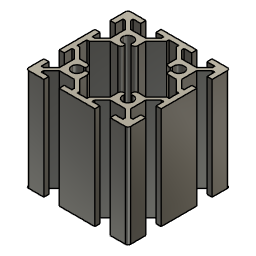
Misumi 4040 Cube (Autodesk Fusion 360 design; units mm, degrees)
Autodesk Fusion 360 part; units mm, degrees
sketch "Sketch1" plane through (0, 0, 0) normal (0, 0, 1) x (1, 0, 0)
  line L0 (-4, 2.9395) -> (-7.0605, 6)
  line L1 (-7.0605, 6) -> (-8, 6)
  line L2 (-8, 6) -> (-8, 3)
  line L3 (-8, 3) -> (-10, 3)
  line L4 (-2.9395, -4) -> (2.9395, -4)
  line L5 (-2.9395, -4) -> (-6, -7.0605)
  line L6 (-6, -7.0605) -> (-6, -8)
  line L7 (-8, -3) -> (-8, -6)
  line L8 (-8, -6) -> (-7.0608, -6)
  line L9 (-7.0608, -6) -> (-4, -2.9392)
  line L10 (-4, -2.9392) -> (-4, 2.9398)
  line L11 (-6, -8) -> (-3, -8)
  line L12 (-9, -10) -> (-3, -10)
  arc A0 (-10, -9) -> (-9, -10) centre (-9, -9) ccw
  line L13 (-10, -9) -> (-10, -3)
  line L14 (-10, -3) -> (-8, -3)
  line L15 (-3, -8) -> (-3, -10)
  line L16 (6, -7.0608) -> (2.9392, -4)
  line L17 (6, -8) -> (6, -7.0608)
  line L18 (3, -8) -> (6, -8)
  line L19 (3, -10) -> (3, -8)
  circle A1 centre (0, 0) radius 2.1
  line L20 (17.0605, -4) -> (14, -7.0605)
  line L21 (14, -7.0605) -> (14, -8)
  line L22 (17, -8) -> (17, -10)
  line L23 (14, -8) -> (17, -8)
  line L24 (24, -2.9395) -> (24, 2.9395)
  line L25 (24, -2.9395) -> (27.0605, -6)
  line L26 (27.0605, -6) -> (28, -6)
  line L27 (28, -6) -> (28, -3)
  line L28 (28, -3) -> (30, -3)
  line L29 (30, -9) -> (30, -3)
  arc A2 (29, -10) -> (30, -9) centre (29, -9) ccw
  line L30 (29, -10) -> (23, -10)
  line L31 (23, -10) -> (23, -8)
  line L32 (23, -8) -> (26, -8)
  line L33 (26, -8) -> (26, -7.0608)
  line L34 (26, -7.0608) -> (22.9392, -4)
  line L35 (22.9392, -4) -> (17.0602, -4)
  line L36 (30, 3) -> (28, 3)
  line L37 (28, 3) -> (28, 6)
  line L38 (28, 6) -> (27.0608, 6)
  line L39 (27.0608, 6) -> (24, 2.9392)
  line L40 (24, 17.0605) -> (27.0605, 14)
  line L41 (27.0605, 14) -> (28, 14)
  line L42 (28, 17) -> (30, 17)
  line L43 (28, 14) -> (28, 17)
  line L44 (22.9395, 24) -> (17.0605, 24)
  line L45 (22.9395, 24) -> (26, 27.0605)
  line L46 (26, 27.0605) -> (26, 28)
  line L47 (26, 28) -> (23, 28)
  line L48 (23, 28) -> (23, 30)
  line L49 (29, 30) -> (23, 30)
  arc A3 (30, 29) -> (29, 30) centre (29, 29) ccw
  line L50 (30, 29) -> (30, 23)
  line L51 (30, 23) -> (28, 23)
  line L52 (28, 23) -> (28, 26)
  line L53 (28, 26) -> (27.0608, 26)
  line L54 (27.0608, 26) -> (24, 22.9392)
  line L55 (24, 22.9392) -> (24, 17.0602)
  line L56 (17, 30) -> (17, 28)
  line L57 (17, 28) -> (14, 28)
  line L58 (14, 28) -> (14, 27.0608)
  line L59 (14, 27.0608) -> (17.0608, 24)
  line L60 (2.9395, 24) -> (6, 27.0605)
  line L61 (6, 27.0605) -> (6, 28)
  line L62 (3, 28) -> (3, 30)
  line L63 (6, 28) -> (3, 28)
  line L64 (-4, 22.9395) -> (-4, 17.0605)
  line L65 (-4, 22.9395) -> (-7.0605, 26)
  line L66 (-7.0605, 26) -> (-8, 26)
  line L67 (-8, 26) -> (-8, 23)
  line L68 (-8, 23) -> (-10, 23)
  line L69 (-10, 29) -> (-10, 23)
  arc A4 (-9, 30) -> (-10, 29) centre (-9, 29) ccw
  line L70 (-9, 30) -> (-3, 30)
  line L71 (-3, 30) -> (-3, 28)
  line L72 (-3, 28) -> (-6, 28)
  line L73 (-6, 28) -> (-6, 27.0608)
  line L74 (-6, 27.0608) -> (-2.9392, 24)
  line L75 (-2.9392, 24) -> (2.9398, 24)
  line L76 (-10, 17) -> (-8, 17)
  line L77 (-8, 17) -> (-8, 14)
  line L78 (-8, 14) -> (-7.0608, 14)
  line L79 (-7.0608, 14) -> (-4, 17.0608)
  line L80 (3, -10) -> (17, -10)
  line L81 (-10, 3) -> (-10, 17)
  line L82 (3, 30) -> (17, 30)
  line L83 (30, 3) -> (30, 17)
  circle A5 centre (20, 0) radius 2.1
  circle A6 centre (20, 20) radius 2.1
  circle A7 centre (0, 20) radius 2.1
  line L84 (4, 2.9392) -> (4, -2.9398) construction
  line L85 (-2.9392, 4) -> (2.9398, 4) construction
  line L86 (2.9398, 4) -> (0.857, 1.9172) construction
  line L87 (4, 2.9392) -> (1.9174, 0.8566) construction
  arc A8 (0.857, 1.9172) -> (0.0003, 4) centre (0.0003, 2.7824) ccw
  line L88 (0, 0) -> (-9, -9) construction
  arc A9 (4, 0.0003) -> (1.9172, 0.857) centre (2.7824, 0.0003) ccw
  line L89 (-2.9392, 4) -> (-7.0605, 8.1213)
  line L90 (-7.0605, 8.1213) -> (-8, 8.1213)
  line L91 (-8, 8.1213) -> (-8, 11.8787)
  line L92 (8.1213, -7.0605) -> (8.1213, -8)
  line L93 (4, -2.9392) -> (8.1213, -7.0605)
  line L94 (-2.9392, 4) -> (0.0003, 4)
  line L95 (4, 0.0003) -> (4, -2.9398)
  arc A10 (19.9997, 4) -> (19.143, 1.9172) centre (19.9997, 2.7824) ccw
  line L96 (19.9997, 4) -> (22.9398, 4)
  line L97 (16, -2.9392) -> (16, 0.0003)
  arc A11 (18.0828, 0.857) -> (16, 0.0003) centre (17.2176, 0.0003) ccw
  line L98 (27.0605, 8.1213) -> (28, 8.1213)
  line L99 (22.9392, 4) -> (27.0605, 8.1213)
  line L100 (11.8787, -7.0605) -> (11.8787, -8)
  line L101 (11.8787, -8) -> (8.1213, -8)
  line L102 (16, -2.9392) -> (11.8787, -7.0605)
  arc A12 (16, 19.9997) -> (18.0828, 19.143) centre (17.2176, 19.9997) ccw
  line L103 (16, 19.9997) -> (16, 22.9398)
  line L104 (22.9392, 16) -> (19.9997, 16)
  arc A13 (19.143, 18.0828) -> (19.9997, 16) centre (19.9997, 17.2176) ccw
  line L105 (11.8787, 27.0605) -> (11.8787, 28)
  line L106 (16, 22.9392) -> (11.8787, 27.0605)
  line L107 (27.0605, 11.8787) -> (28, 11.8787)
  line L108 (28, 11.8787) -> (28, 8.1213)
  line L109 (22.9392, 16) -> (27.0605, 11.8787)
  arc A14 (0.0003, 16) -> (0.857, 18.0828) centre (0.0003, 17.2176) ccw
  line L110 (0.0003, 16) -> (-2.9398, 16)
  line L111 (4, 22.9392) -> (4, 19.9997)
  arc A15 (1.9172, 19.143) -> (4, 19.9997) centre (2.7824, 19.9997) ccw
  line L112 (-7.0605, 11.8787) -> (-8, 11.8787)
  line L113 (-2.9392, 16) -> (-7.0605, 11.8787)
  line L114 (8.1213, 27.0605) -> (8.1213, 28)
  line L115 (8.1213, 28) -> (11.8787, 28)
  line L116 (4, 22.9392) -> (8.1213, 27.0605)
  arc A16 (0.5376, 2.03) -> (1.1291, 2.3259) centre (0.6656, 2.5134) ccw
  arc A17 (2.3259, 1.1291) -> (2.03, 0.5376) centre (2.5134, 0.6656) ccw
  arc A18 (17.97, 0.5376) -> (17.6741, 1.1291) centre (17.4866, 0.6656) ccw
  arc A19 (18.8709, 2.3259) -> (19.4624, 2.03) centre (19.3344, 2.5134) ccw
  arc A20 (19.4624, 17.97) -> (18.8709, 17.6741) centre (19.3344, 17.4866) ccw
  arc A21 (17.6741, 18.8709) -> (17.97, 19.4624) centre (17.4866, 19.3344) ccw
  arc A22 (2.03, 19.4624) -> (2.3259, 18.8709) centre (2.5134, 19.3344) ccw
  arc A23 (1.1291, 17.6741) -> (0.5376, 17.97) centre (0.6656, 17.4866) ccw
  point P0 (10, 10)
  dimension "d6" = 10
  dimension "d7" = 10
  dimension "d9" = 360
  dimension "d12" = 360
  dimension "d13" = 0.5
  constraint coincident L19.start L80.start
  constraint coincident L3.end L81.start
  constraint coincident L85.end L86.start
  constraint parallel L9 L86
  constraint coincident L84.start L87.start
  constraint coincident A1 L87.end
  constraint parallel L86 L87
  constraint tangent L85 A8
  constraint coincident L85 A8.end
  constraint coincident L86 A8.start
  constraint midpoint L85 A8.end
  constraint coincident A1 L86.end
  constraint coincident A1.centre L88.start
  constraint coincident A0.centre L88.end
  constraint symmetric L86.end L88 A9.end
  constraint symmetric A8.end L88 A9.start
  constraint symmetric A8 L88 A9
  constraint coincident L85.start L89.start
  constraint parallel L0 L89
  constraint perpendicular L81 L90
  constraint perpendicular L90 L91
  constraint coincident L1.end L91
  constraint equal L1 L90
  constraint symmetric L88 L85.start L93.start
  constraint symmetric L88 L89.end L92.start
  constraint symmetric L88 L90.end L92.end
  constraint coincident L84.end L95.end
  constraint coincident L91.end L112.end
  constraint tangent A1 A16
  constraint coincident A8 A16.end
  constraint coincident A1 A16.start
  constraint tangent A8 A16
  constraint symmetric L88 A16.start A17.end
  constraint symmetric L88 A16.end A17.start
  constraint symmetric L88 A16 A17
  measures "d6" horizontal distance of A1.centre P0
  measures "d7" vertical distance of A1.centre P0
  measures "d13" radius of A16
extrude "Extrude1" add sketch "Sketch1" along normal blind 40
equation "Length = 40 mm"
equation "d7 = d6"
equation "d14 = Length"
